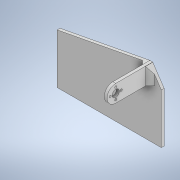
# Autodesk Inventor part: gripperMove
Saved by Autodesk Inventor 2020 (Build 240168000, 168)
## iProperties
Created: 2019-12-27
Part Number: gripperMove
Material: Generic
Document SubType Name: Modeling
Designer: tdmp4
Density: 1 g/cm^3
Appearance: Default
Author: tdmp4
Autodesk Inventor part; units mm, degrees
ref_plane "YZ Plane" through (0, 0, 0) normal (1, 0, 0) x (0, 1, 0)
ref_plane "XZ Plane" through (0, 0, 0) normal (0, 1, 0) x (-1, 0, 0)
ref_plane "XY Plane" through (0, 0, 0) normal (0, 0, 1) x (1, 0, 0)
sketch "Sketch1" plane through (0, 0, 0) normal (1, 0, 0) x (0, 1, 0)
  circle A0 centre (0, 0) radius 15.24
  circle A1 centre (0, 0) radius 6.35
  circle A2 centre (9.779, 0) radius 1.7859
  circle A3 centre (0, -9.779) radius 1.7859
  circle A4 centre (-9.779, 0) radius 1.7859
  circle A5 centre (0, 9.779) radius 1.7859
  dimension "d0" = 30.48
  dimension "d2" = 12.7
  dimension "d3" = 3.5719
  dimension "d4" = 3.5719
  dimension "d5" = 3.5719
  dimension "d6" = 3.5719
  constraints: 6 centre point, 1 coincident
  measures "d0" diameter of A0
  measures "d2" diameter of A1
  measures "d3" diameter of A2
  measures "d4" diameter of A3
  measures "d5" diameter of A4
  measures "d6" diameter of A5
extrude "Extrusion1" add sketch "Sketch1" along normal blind 5.08
sketch "Sketch2" plane through (5.08, 0, 0) normal (1, 0, 0) x (0, 0, -1)
  circle A0 centre (0, 0) radius 15.24 projected
  arc A1 (0, -15.24) -> (0, 15.24) centre (0, 0) ccw
  line L0 (0, 15.24) -> (60.96, 15.24)
  line L1 (60.96, 15.24) -> (60.96, -15.24)
  line L2 (60.96, -15.24) -> (0, -15.24)
  line L3 (60.96, -15.24) -> (66.04, -15.24)
  line L4 (66.04, -15.24) -> (60.96, 15.24)
  line L5 (60.96, 15.24) -> (66.04, 15.24)
  line L6 (66.04, 15.24) -> (66.04, -15.24)
  dimension "d9" = 60.96
  dimension "d10" = 30.48
  dimension "d11" = 5.08
  dimension "d19" = 5.08
  constraints: 14 end point, 4 point on circle, 2 horizontal, 2 perpendicular, 1 centre point, 1 point on line
  measures "d9" distance of L0.start L0.end
  measures "d10" distance of L0.end L1.end
  measures "d11" distance of L1.end L3.end
  measures "d19" distance of L0.end L5.end
extrude "Extrusion2" add sketch "Sketch2" against normal blind 5.08 contours A0 L0 L1 L2 | L4 L3 L1 | L5 L6 L4
sketch "Sketch3" plane through (5.08, -15.24, -66.04) normal (0, -1, 0) x (1, 0, 0)
  line L0 (0, 0) -> (-5.08, 0) projected
  line L1 (0, 0) -> (-165.1, 0)
  line L2 (-165.1, 0) -> (-165.1, 5.08)
  line L3 (-165.1, 5.08) -> (0, 5.08)
  line L4 (0, 5.08) -> (0, 0)
  line L5 (-5.08, 0) -> (20.32, 0)
  line L6 (20.32, 0) -> (20.32, 5.08)
  line L7 (20.32, 5.08) -> (-5.08, 5.08)
  line L8 (-5.08, 5.08) -> (-5.08, 0)
  point P0 (-5.08, 66.04)
  point P1 (0, 5.08)
  dimension "d14" = 165.1
  dimension "d15" = 5.08
  dimension "d16" = 25.4
  constraints: 16 end point, 4 parallel, 2 horizontal, 2 perpendicular
  measures "d14" distance of L2.end L3.end
  measures "d15" distance of L1.end L2.end
  measures "d16" distance of L7.end L6.end
extrude "Extrusion3" add sketch "Sketch3" along normal blind 88.9
sketch "Sketch4" plane through (0, -15.24, -66.04) normal (0, 0, -1) x (-1, 0, 0)
  line L0 (-25.4, 0) -> (-25.4, -88.9) projected
  line L1 (0, 0) -> (160.02, 0) projected
  line L2 (0, 30.48) -> (160.02, 0)
  line L3 (160.02, 0) -> (0, 0)
  line L4 (0, 0) -> (0, 30.48)
  line L5 (-5.08, 30.1221) -> (-25.4, 0)
  line L6 (-5.08, 30.1221) -> (-5.08, 0)
  line L7 (-25.4, 0) -> (-5.08, 0) projected
  line L8 (-5.08, 0) -> (-25.4, 0)
  point P0 (0, 15.24)
  constraints: 12 end point, 2 perpendicular, 1 collinear, 1 vertical
extrude "Extrusion4" add sketch "Sketch4" against normal blind 5.08
chamfer "Chamfer1" distance 7.9375 angle 45 1 edges at (5.08, -0.1789, -60.96)
chamfer "Chamfer2" distance 7.9375 angle 45 1 edges at (0, 0, -60.96)
sketch "Sketch5" plane through (25.4, -104.14, -66.04) normal (0, 0, -1) x (-1, 0, 0)
  line L0 (174.7065, 82.6913) -> (4.5265, 82.6913)
  line L1 (4.5265, 82.6913) -> (4.5265, 69.9913)
  line L2 (4.5265, 69.9913) -> (174.7065, 69.9913)
  line L3 (174.7065, 69.9913) -> (174.7065, 82.6913)
  line L4 (174.7065, 57.279) -> (4.5265, 57.279)
  line L5 (4.5265, 57.279) -> (4.5265, 44.579)
  line L6 (4.5265, 44.579) -> (174.7065, 44.579)
  line L7 (174.7065, 44.579) -> (174.7065, 57.279)
  line L8 (174.7065, 33.5337) -> (4.5265, 33.5337)
  line L9 (4.5265, 33.5337) -> (4.5265, 20.8337)
  line L10 (4.5265, 20.8337) -> (174.7065, 20.8337)
  line L11 (174.7065, 20.8337) -> (174.7065, 33.5337)
  line L12 (132.138, 94.0344) -> (119.438, 94.0344)
  line L13 (119.438, 94.0344) -> (119.438, 5.1344)
  line L14 (119.438, 5.1344) -> (132.138, 5.1344)
  line L15 (132.138, 5.1344) -> (132.138, 94.0344)
  line L16 (36.8203, 108.1081) -> (24.1203, 108.1081)
  line L17 (24.1203, 108.1081) -> (24.1203, 6.5081)
  line L18 (24.1203, 6.5081) -> (36.8203, 6.5081)
  line L19 (36.8203, 6.5081) -> (36.8203, 108.1081)
  point P0 (25.4, 104.14)
  point P1 (132.138, 69.9913)
  point P2 (132.138, 82.6913)
  point P3 (119.438, 82.6913)
  point P4 (36.8203, 82.6913)
  point P5 (24.1203, 82.6913)
  point P6 (24.1203, 69.9913)
  point P7 (24.1203, 57.279)
  point P8 (24.1203, 44.579)
  point P9 (24.1203, 33.5337)
  point P10 (24.1203, 20.8337)
  point P11 (36.8203, 20.8337)
  point P12 (119.438, 20.8337)
  point P13 (132.138, 20.8337)
  point P14 (132.138, 33.5337)
  point P15 (132.138, 44.579)
  point P16 (132.138, 57.279)
  point P17 (119.438, 44.579)
  point P18 (119.438, 33.5337)
  point P19 (36.8203, 33.5337)
  point P20 (36.8203, 44.579)
  point P21 (119.438, 69.9913)
  point P22 (119.438, 57.279)
  point P23 (36.8203, 57.279)
  point P24 (36.8203, 69.9913)
  dimension "d28" = 12.7
  dimension "d29" = 170.18
  dimension "d30" = 12.7
  dimension "d31" = 12.7
  dimension "d32" = 12.7
  dimension "d33" = 88.9
  dimension "d34" = 12.7
  dimension "d35" = 101.6
  constraints: 40 end point, 10 parallel, 5 horizontal, 5 perpendicular
  measures "d28" distance of L0.end L1.end
  measures "d29" distance of L0.start L0.end
  measures "d30" distance of L4.end L5.end
  measures "d31" distance of L8.end L9.end
  measures "d32" distance of L13.end L14.end
  measures "d33" distance of L14.end L12.start
  measures "d34" distance of L18.end L17.end
  measures "d35" distance of L18.end L16.start
extrude "Extrusion5" add sketch "Sketch5" along normal blind 2.54 contours L3 L2 L15 L0 | L15 L2 L13 L0 | L0 L13 L12 L15 | L13 L2 L19 L0 | L15 L4 L13 L2 | L19 L2 L17 L0 | L0 L17 L16 L19 | L15 L6 L13 L4 | L4 L7 L6 L15 | L17 L2 L1 L0 | L19 L4 L17 L2 | L13 L6 L19 L4 | L15 L8 L13 L6 | L19 L6 L17 L4 | L15 L10 L13 L8 | L8 L11 L10 L15 | L17 L6 L5 L4 | L19 L8 L17 L6 | L13 L10 L19 L8 | L15 L14 L13 L10 | L19 L10 L17 L8 | L17 L10 L9 L8 | L19 L18 L17 L10
body "Solid1"
